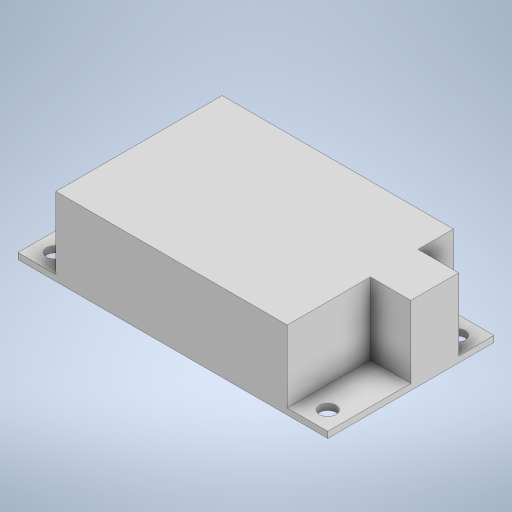
# Autodesk Inventor part: 5V
Saved by Autodesk Inventor 2023 (Build 270158000, 158)
## iProperties
Created: 2022-04-18
Part Number: 5V
Material: Generic
Document SubType Name: Modeling
Designer: benni
Density: 1 g/cm^3
Appearance: Default
Author: benni
Autodesk Inventor part; units mm, degrees
ref_plane "YZ Plane" through (0, 0, 0) normal (1, 0, 0) x (0, 1, 0)
ref_plane "XZ Plane" through (0, 0, 0) normal (0, 1, 0) x (-1, 0, 0)
ref_plane "XY Plane" through (0, 0, 0) normal (0, 0, 1) x (1, 0, 0)
sketch "Sketch1" plane through (0, 0, 0) normal (0, 1, 0) x (-1, 0, 0)
  line L0 (0, 0) -> (75.5, 0)
  line L1 (75.5, 0) -> (75.5, -40.5)
  line L2 (75.5, -40.5) -> (0, -40.5)
  line L3 (0, -40.5) -> (0, 0)
  line L4 (75.5, -20.25) -> (0, -20.25)
  line L5 (37.75, -40.5) -> (37.75, 0)
  circle A0 centre (71, -36) radius 2
  circle A1 centre (4.5, -36) radius 2
  circle A2 centre (71, -4.5) radius 2
  circle A3 centre (4.5, -4.5) radius 2
  dimension "d0" = 75.5
  dimension "d1" = 40.5
  dimension "d2" = 31.5
  dimension "d3" = 66.5
  dimension "d4" = 4
  constraints: 12 end point, 4 centre point, 4 midpoint, 3 symmetric about line, 2 parallel, 1 coincident, 1 horizontal, 1 perpendicular, 3 other
  measures "d0" distance of L1.end L2.end
  measures "d1" distance of L0.end L1.end
  measures "d2" diameter of point (71, -36) L4
  measures "d3" diameter of point (71, -36) L5
  measures "d4" diameter of A0
extrude "Extrusion1" add sketch "Sketch1" along normal blind 1.5
sketch "Sketch2" plane through (0, 1.5, 0) normal (0, 1, 0) x (1, 0, 0)
  line L0 (0, 40.5) -> (-75.5, 40.5) projected
  line L1 (-75.5, 0) -> (0, 0) projected
  line L2 (-66.2537, 40.5) -> (-9.8709, 40.5)
  line L3 (-9.8709, 40.5) -> (-9.8709, 0)
  line L4 (-9.8709, 0) -> (-66.2537, 0)
  line L5 (-66.2537, 0) -> (-66.2537, 40.5)
  line L6 (0, 0) -> (0, 40.5) projected
  line L7 (-9.8709, 31.9029) -> (0, 31.9029)
  line L8 (0, 31.9029) -> (0, 20.25)
  line L9 (0, 20.25) -> (-9.8709, 20.25)
  line L10 (-9.8709, 20.25) -> (-9.8709, 31.9029)
  constraints: 16 end point, 4 parallel, 3 point on line, 2 horizontal, 2 perpendicular, 1 midpoint
extrude "Extrusion2" add sketch "Sketch2" along normal blind 17.5 contours L3 L1 L5 L0 | L6 L9 L3 L7
body "Solid1"
